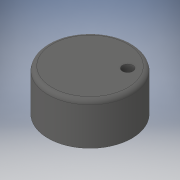
# Autodesk Inventor part: Hub
Saved by Autodesk Inventor 2017 (Build 210142000, 142)
## iProperties
Part Number: Hub
Material: ABS-Kunststoff
Document SubType Name: Modeling
Designer: OleSi
Density: 1.06 g/cm^3
Appearance: Grau
Author: OleSi
Autodesk Inventor part; units mm, degrees
ref_plane "YZ Plane" through (0, 0, 0) normal (1, 0, 0) x (0, 1, 0)
ref_plane "XZ Plane" through (0, 0, 0) normal (0, 1, 0) x (-1, 0, 0)
ref_plane "XY Plane" through (0, 0, 0) normal (0, 0, 1) x (1, 0, 0)
sketch "Skizze1" plane through (0, 0, 0) normal (0, 0, 1) x (1, 0, 0)
  circle A0 centre (0, 0) radius 20
  dimension "d0" = 40
  constraints: 1 centre point, 1 coincident
  measures "d0" diameter of A0
extrude "Extrusion1" add sketch "Skizze1" along normal blind 20
fillet "Rundung1" radius 2 1 edges at (-20, 0, 20)
sketch "Skizze2" plane through (0, 0, 20) normal (0, 0, 1) x (1, 0, 0)
  circle A0 centre (10, 8) radius 3.75
  point P0 (0, 0)
  dimension "d4" = 7.5
  constraints: 1 centre point
  measures "d4" diameter of A0
hole "Bohrung1" at (10, 8, 20) direction (0, 0, -1) diameter 5 end through all
sketch "Skizze3" plane through (0, 0, 0) normal (0, 0, -1) x (-1, 0, 0)
  circle A0 centre (0, 0) radius 2.5
  circle A1 centre (0, 0) radius 2
  dimension "d12" = 5
  dimension "d13" = 4
  constraints: 2 centre point, 2 coincident
  measures "d12" diameter of A0
  measures "d13" diameter of A1
extrude "Extrusion2" cut sketch "Skizze3" against normal blind 0.5
